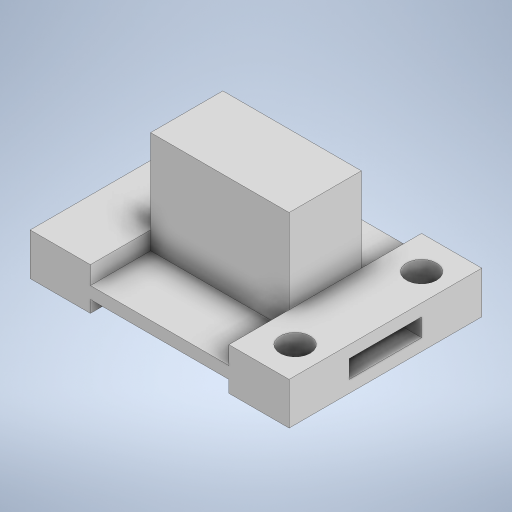
# Autodesk Inventor part: Langbektang houder
Saved by Autodesk Inventor 2023.2 (Build 272271000, 271)
## iProperties
Created: 2020-09-09
Part Number: Langbektang houder
Material: Generic
Document SubType Name: Modeling
Designer: nathan.bollaert
Density: 1 g/cm^3
Appearance: Default
Author: nathan.bollaert
Autodesk Inventor part; units mm, degrees
ref_plane "YZ Plane" through (0, 0, 0) normal (1, 0, 0) x (0, 1, 0)
ref_plane "XZ Plane" through (0, 0, 0) normal (0, 1, 0) x (-1, 0, 0)
ref_plane "XY Plane" through (0, 0, 0) normal (0, 0, 1) x (1, 0, 0)
sketch "Sketch1" plane through (0, 0, 0) normal (0, 1, 0) x (-1, 0, 0)
  line L0 (0, 0) -> (31, 0)
  line L1 (31, 0) -> (31, -12)
  line L2 (31, -12) -> (0, -12)
  line L3 (0, -12) -> (0, 0)
  line L4 (4, -12) -> (27, -12)
  line L5 (27, -12) -> (27, 0)
  line L6 (27, 0) -> (4, 0)
  line L7 (4, 0) -> (4, -12)
  point P0 (27, 0)
  point P1 (4, 0)
  dimension "d230" = 31
  dimension "d231" = 12
  dimension "d232" = 23
  dimension "d234" = 4
  constraints: 16 end point, 5 parallel, 2 horizontal, 2 perpendicular, 1 point on line
  measures "d230" distance of L1.end L2.end
  measures "d231" distance of L0.end L1.end
  measures "d232" distance of L6.end L5.end
  measures "d234" distance from line of L7 L2.end
extrude "Extrusion1" add sketch "Sketch1" along normal blind 3 contours L0 L7 L2 L3 | L0 L1 L2 L5
extrude "Extrusion2" add sketch "Sketch1" along normal blind 19 and the other way blind 4 contours L0 L5 L2 L7
sketch "Sketch2" plane through (0, 3, 0) normal (0, 1, 0) x (1, 0, 0)
  line L0 (-27, -10) -> (-37, -10)
  line L1 (-37, -10) -> (-37, 22)
  line L2 (-37, 22) -> (-27, 22)
  line L3 (-27, 22) -> (-27, -10)
  line L4 (-27, 12) -> (-27, 0) projected
  line L5 (-4, 22) -> (6, 22)
  line L6 (6, 22) -> (6, -10)
  line L7 (6, -10) -> (-4, -10)
  line L8 (-4, -10) -> (-4, 22)
  line L9 (-4, 0) -> (-4, 12) projected
  point P0 (0, 0)
  point P1 (-27, 6)
  point P2 (-27, 6)
  point P3 (-27, 6)
  point P4 (-4, 6)
  point P5 (-4, 6)
  point P6 (-4, 6)
  dimension "d241" = 10
  dimension "d242" = 32
  dimension "d243" = 10
  dimension "d244" = 32
  constraints: 16 end point, 6 midpoint, 4 coincident, 4 parallel, 2 horizontal, 2 perpendicular
  measures "d241" distance of L1.end L2.end
  measures "d242" distance of L0.end L1.end
  measures "d243" distance of L6.end L7.end
  measures "d244" distance of L5.end L6.end
extrude "Extrusion3" add sketch "Sketch2" along normal blind 2
sketch "Sketch3" plane through (0, 0, 0) normal (0, -1, 0) x (1, 0, 0)
  line L0 (-37, -22) -> (-37, 10) projected
  line L1 (-27, -12) -> (-27, -22) projected
  line L2 (-37, 10) -> (-27, 10)
  line L3 (-27, 10) -> (-27, -22)
  line L4 (-27, -22) -> (-37, -22)
  line L5 (-37, -22) -> (-37, 10)
  line L6 (6, -22) -> (-4, -22) projected
  line L7 (6, 10) -> (6, -22) projected
  line L8 (-4, -22) -> (6, -22)
  line L9 (6, -22) -> (6, 10)
  line L10 (6, 10) -> (-4, 10)
  line L11 (-4, 10) -> (-4, -22)
  point P0 (0, 0)
  constraints: 16 end point, 4 parallel, 2 horizontal, 2 perpendicular
extrude "Extrusion4" add sketch "Sketch3" along normal blind 2
sketch "Sketch4" plane through (0, 0, 0) normal (0, 1, 0) x (1, 0, 0)
  line L0 (-4, 22) -> (-4, 12) projected
  line L1 (6, -10) -> (-4, -10)
  line L2 (-4, 22) -> (6, 22)
  line L3 (-27, 22) -> (-37, 22) projected
  line L4 (-27, 22) -> (-37, 22)
  line L5 (-37, 22) -> (-37, -10)
  line L6 (-37, -10) -> (-27, -10)
  line L7 (-4, 0) -> (-27, 0) projected
  line L8 (6, -10) -> (-4, -10)
  line L9 (-4, -10) -> (-4, 0)
  line L10 (-4, 0) -> (6, 0)
  line L11 (6, 0) -> (6, -10)
  line L12 (-27, -10) -> (-37, -10)
  line L13 (-37, -10) -> (-37, 0)
  line L14 (-37, 0) -> (-27, 0)
  line L15 (-27, 0) -> (-27, -10)
  line L16 (-27, 12) -> (-37, 12)
  line L17 (-37, 12) -> (-37, 22)
  line L18 (-37, 22) -> (-27, 22)
  line L19 (-27, 22) -> (-27, 12)
  line L20 (0, 12) -> (-4, 12) projected
  line L21 (-4, 22) -> (6, 22) projected
  line L22 (-4, 12) -> (6, 12)
  line L23 (6, 12) -> (6, 22)
  line L24 (6, 22) -> (-4, 22)
  line L25 (-4, 22) -> (-4, 12)
  line L26 (-37, 22) -> (-37, -10) projected
  line L27 (-37, 22) -> (6, 22)
  line L28 (6, 22) -> (6, 12)
  line L29 (6, 12) -> (-37, 12)
  line L30 (-37, 12) -> (-37, 22)
  line L31 (6, -10) -> (-37, -10)
  line L32 (-37, -10) -> (-37, 0)
  line L33 (-37, 0) -> (6, 0)
  line L34 (6, 0) -> (6, -10)
  point P0 (0, 0)
  constraints: 58 end point, 14 parallel, 8 horizontal, 7 perpendicular, 2 point on line
extrude "Extrusion5" add sketch "Sketch4" along normal blind 3 contours L2 L23 L22 L20 L0 | L19 L16 L5 L3 | L1 L9 L10 L11 | L6 L5 L14 L15
extrude "Extrusion6" add sketch "Sketch4" along normal blind 2
sketch "Sketch5" plane through (0, -4, 0) normal (0, -1, 0) x (1, 0, 0)
  circle A0 centre (-21, -6) radius 6
  line L0 (-4, 0) -> (-27, 0) projected
  line L1 (-27, 0) -> (-27, -12) projected
  point P0 (0, 0)
  dimension "d255" = 12
  dimension "d256" = 6
  dimension "d257" = 6
  constraints: 1 centre point
  measures "d255" diameter of A0
  measures "d256" distance from line of L0 A0.centre
  measures "d257" distance from line of L1 A0.centre
extrude "Extrusion7" add sketch "Sketch5" along normal blind 4 contours A0
sketch "Sketch6" plane through (-21, -8, -6) normal (0, -1, 0) x (1, 0, 0)
  circle A0 centre (0, 0) radius 2.5
  circle A1 centre (0, 0) radius 6 projected
  point P0 (21, 6)
  dimension "d260" = 5
  dimension "d261" = 3.5
  constraints: 1 centre point
  measures "d260" diameter of A0
  measures "d261" radial gap between concentric circles of A1 A0
extrude "Extrusion8" add sketch "Sketch6" along normal blind 3 contours A0
sketch "Sketch7" plane through (-21, -11, -6) normal (0, -1, 0) x (1, 0, 0)
  line L0 (-6, -6) -> (0, -6) projected
  line L1 (-6, 6) -> (-6, 0) projected
  circle A0 centre (0, 0) radius 1
  point P0 (21, 6)
  dimension "d266" = 2
  dimension "d267" = 6
  dimension "d268" = 6
  constraints: 1 centre point
  measures "d266" diameter of A0
  measures "d267" distance from line of L1 A0.centre
  measures "d268" distance from line of L0 A0.centre
extrude "Extrusion9" cut sketch "Sketch7" against normal blind 6
sketch "Sketch22" plane through (0, 5, 0) normal (0, 1, 0) x (1, 0, 0)
  circle A0 centre (1.5, -4.5) radius 2.5
  circle A1 centre (1.5, 16.5) radius 2.5
  line L0 (-4, 22) -> (-4, 12) projected
  line L1 (-4, 0) -> (-4, 12) projected
  line L2 (-27, 0) -> (-27, 6) projected
  line L3 (-4, 6) -> (-27, 6)
  point P0 (0, 0)
  dimension "d271" = 5
  dimension "d272" = 5
  dimension "d273" = 21
  dimension "d274" = 5.5
  constraints: 2 centre point, 2 end point, 1 horizontal, 1 midpoint, 1 symmetric about line, 1 vertical alignment
  measures "d271" diameter of A0
  measures "d272" diameter of A1
  measures "d273" distance of A0.centre A1.centre
  measures "d274" distance from line of L0 A1.centre
extrude "Extrusion26" cut sketch "Sketch22" against normal blind 8
body "Solid5"
